Autodesk Fusion 360 part; units mm, degrees
note: some values were not read from the file. Set by a fixed rule: which sketch regions a step uses.
(part 3 of 10)
  spline S13 degree 5 poles (-8.3931, 13.6219) (-8.3929, 13.6198) (-8.3924, 13.6155) (-8.3916, 13.6092) (-8.3906, 13.6008) (-8.3893, 13.5903) (-8.3879, 13.5798) (-8.3866, 13.5693) (-8.3853, 13.5589) (-8.3839, 13.5485) (-8.3826, 13.5382) (-8.3812, 13.5278) (-8.3798, 13.5175) (-8.3784, 13.5072) (-8.377, 13.497) (-8.3755, 13.4867) (-8.3741, 13.4766) (-8.3726, 13.4664) (-8.3712, 13.4563) (-8.3697, 13.4461) (-8.3682, 13.4361) (-8.3667, 13.426) (-8.3652, 13.416) (-8.3637, 13.406) (-8.3621, 13.396) (-8.3606, 13.3861) (-8.359, 13.3762) (-8.3574, 13.3663) (-8.3558, 13.3565) (-8.3542, 13.3467) (-8.3526, 13.3369) (-8.351, 13.3272) (-8.3494, 13.3174) (-8.3477, 13.3078) (-8.3461, 13.2981) (-8.3444, 13.2885) (-8.3427, 13.2789) (-8.341, 13.2693) (-8.3393, 13.2598) (-8.3376, 13.2503) (-8.3359, 13.2408) (-8.3342, 13.2313) (-8.3324, 13.2219) (-8.3307, 13.2125) (-8.3289, 13.2032) (-8.3271, 13.1939) (-8.3254, 13.1846) (-8.3236, 13.1753) (-8.3218, 13.1661) (-8.3199, 13.1569) (-8.3181, 13.1478) (-8.3163, 13.1386) (-8.3145, 13.1296) (-8.3126, 13.1205) (-8.3107, 13.1115) (-8.3089, 13.1025) (-8.307, 13.0935) (-8.3051, 13.0846) (-8.3032, 13.0757) (-8.3013, 13.0668) (-8.2994, 13.058) (-8.2975, 13.0492) (-8.2956, 13.0404) (-8.2936, 13.0317) (-8.2917, 13.023) (-8.2897, 13.0143) (-8.2878, 13.0057) (-8.2858, 12.9971) (-8.2838, 12.9885) (-8.2818, 12.98) (-8.2799, 12.9715) (-8.2779, 12.963) (-8.2759, 12.9546) (-8.2738, 12.9462) (-8.2718, 12.9379) (-8.2698, 12.9295) (-8.2678, 12.9212) (-8.2657, 12.913) (-8.2637, 12.9048) (-8.2616, 12.8966) (-8.2596, 12.8884) (-8.2575, 12.8803) (-8.2554, 12.8722) (-8.2534, 12.8642) (-8.2513, 12.8562) (-8.2492, 12.8482) (-8.2471, 12.8403) (-8.245, 12.8324) (-8.2429, 12.8245) (-8.2408, 12.8167) (-8.2387, 12.8089) (-8.2366, 12.8011) (-8.2345, 12.7934) (-8.2323, 12.7857) (-8.2302, 12.7781) (-8.2281, 12.7705) (-8.2259, 12.7629) (-8.2238, 12.7554) (-8.2216, 12.7479) (-8.2195, 12.7404) (-8.2173, 12.733) (-8.2152, 12.7256) (-8.213, 12.7183) (-8.2109, 12.711) (-8.2087, 12.7037) (-8.2065, 12.6965) (-8.2044, 12.6893) (-8.2022, 12.6821) (-8.2, 12.675) (-8.1978, 12.6679) (-8.1956, 12.6609) (-8.1935, 12.6539) (-8.1913, 12.6469) (-8.1891, 12.64) (-8.1869, 12.6331) (-8.1847, 12.6263) (-8.1825, 12.6195) (-8.1803, 12.6127) (-8.1782, 12.606) (-8.176, 12.5993) (-8.1738, 12.5926) (-8.1716, 12.586) (-8.1694, 12.5795) (-8.1672, 12.5729) (-8.165, 12.5665) (-8.1628, 12.56) (-8.1606, 12.5536) (-8.1584, 12.5473) (-8.1563, 12.5409) (-8.1541, 12.5347) (-8.1519, 12.5284) (-8.1497, 12.5222) (-8.1475, 12.5161) (-8.1453, 12.51) (-8.1432, 12.5039) (-8.141, 12.4979) (-8.1388, 12.4919) (-8.1366, 12.4859) (-8.1345, 12.48) (-8.1323, 12.4742) (-8.1302, 12.4683) (-8.128, 12.4626) (-8.1258, 12.4568) (-8.1237, 12.4512) (-8.1215, 12.4455) (-8.1194, 12.4399) (-8.1173, 12.4344) (-8.1151, 12.4289) (-8.113, 12.4234) (-8.1109, 12.418) (-8.1088, 12.4126) (-8.1067, 12.4073) (-8.1046, 12.402) (-8.1025, 12.3967) (-8.1004, 12.3915) (-8.0983, 12.3864) (-8.0962, 12.3813) (-8.0941, 12.3762) (-8.0921, 12.3712) (-8.09, 12.3662) (-8.088, 12.3613) (-8.0859, 12.3564) (-8.0839, 12.3516) (-8.0819, 12.3468) (-8.0799, 12.3421) (-8.0779, 12.3374) (-8.0759, 12.3327) (-8.0739, 12.3281) (-8.0719, 12.3236) (-8.0699, 12.3191) (-8.068, 12.3146) (-8.066, 12.3102) (-8.0641, 12.3059) (-8.0622, 12.3016) (-8.0603, 12.2973) (-8.0584, 12.2931) (-8.0565, 12.289) (-8.0546, 12.2848) (-8.0527, 12.2808) (-8.0509, 12.2768) (-8.0491, 12.2728) (-8.0472, 12.2689) (-8.0454, 12.265) (-8.0436, 12.2612) (-8.0419, 12.2575) (-8.0401, 12.2538) (-8.0383, 12.2501) (-8.0366, 12.2465) (-8.0349, 12.243) (-8.0332, 12.2395) (-8.0315, 12.236) (-8.0298, 12.2326) (-8.0282, 12.2293) (-8.0265, 12.226) (-8.0249, 12.2228) (-8.0233, 12.2196) (-8.0218, 12.2164) (-8.0202, 12.2134) (-8.0187, 12.2104) (-8.0171, 12.2074) (-8.0156, 12.2045) (-8.0142, 12.2016) (-8.0127, 12.1988) (-8.0113, 12.1961) (-8.0098, 12.1934) (-8.0084, 12.1908) (-8.0071, 12.1882) (-8.0057, 12.1857) (-8.0044, 12.1832) (-8.0031, 12.1808) (-8.0018, 12.1785) (-8.0006, 12.1762) (-7.9994, 12.1739) (-7.9982, 12.1718) (-7.997, 12.1696) (-7.9958, 12.1676) (-7.9947, 12.1656) (-7.9936, 12.1637) (-7.9926, 12.1618) (-7.9915, 12.16) (-7.9905, 12.1582) (-7.9896, 12.1565) (-7.9886, 12.1549) (-7.9877, 12.1533) (-7.9868, 12.1518) (-7.986, 12.1504) (-7.9852, 12.149) (-7.9844, 12.1477) (-7.9836, 12.1464) (-7.9829, 12.1452) (-7.9823, 12.1441) (-7.9816, 12.1431) (-7.981, 12.1421) (-7.9804, 12.1411) (-7.9799, 12.1403) (-7.9794, 12.1395) (-7.979, 12.1388) (-7.9786, 12.1381) (-7.9782, 12.1375) (-7.9779, 12.137) (-7.9776, 12.1365) (-7.9774, 12.1362) (-7.9772, 12.136) (-7.9772, 12.1359) (-7.9771, 12.1359) knots -1 -1 -1 -1 -1 -1 -0.99583333 -0.99166667 -0.9875 -0.98333333 -0.97916667 -0.975 -0.97083333 -0.96666667 -0.9625 -0.95833333 -0.95416667 -0.95 -0.94583333 -0.94166667 -0.9375 -0.93333333 -0.92916667 -0.925 -0.92083333 -0.91666667 -0.9125 -0.90833333 -0.90416667 -0.9 -0.89583333 -0.89166667 -0.8875 -0.88333333 -0.87916667 -0.875 -0.87083333 -0.86666667 -0.8625 -0.85833333 -0.85416667 -0.85 -0.84583333 -0.84166667 -0.8375 -0.83333333 -0.82916667 -0.825 -0.82083333 -0.81666667 -0.8125 -0.80833333 -0.80416667 -0.8 -0.79583333 -0.79166667 -0.7875 -0.78333333 -0.77916667 -0.775 -0.77083333 -0.76666667 -0.7625 -0.75833333 -0.75416667 -0.75 -0.74583333 -0.74166667 -0.7375 -0.73333333 -0.72916667 -0.725 -0.72083333 -0.71666667 -0.7125 -0.70833333 -0.70416667 -0.7 -0.69583333 -0.69166667 -0.6875 -0.68333333 -0.67916667 -0.675 -0.67083333 -0.66666667 -0.6625 -0.65833333 -0.65416667 -0.65 -0.64583333 -0.64166667 -0.6375 -0.63333333 -0.62916667 -0.625 -0.62083333 -0.61666667 -0.6125 -0.60833333 -0.60416667 -0.6 -0.59583333 -0.59166667 -0.5875 -0.58333333 -0.57916667 -0.575 -0.57083333 -0.56666667 -0.5625 -0.55833333 -0.55416667 -0.55 -0.54583333 -0.54166667 -0.5375 -0.53333333 -0.52916667 -0.525 -0.52083333 -0.51666667 -0.5125 -0.50833333 -0.50416667 -0.5 -0.49583333 -0.49166667 -0.4875 -0.48333333 -0.47916667 -0.475 -0.47083333 -0.46666667 -0.4625 -0.45833333 -0.45416667 -0.45 -0.44583333 -0.44166667 -0.4375 -0.43333333 -0.42916667 -0.425 -0.42083333 -0.41666667 -0.4125 -0.40833333 -0.40416667 -0.4 -0.39583333 -0.39166667 -0.3875 -0.38333333 -0.37916667 -0.375 -0.37083333 -0.36666667 -0.3625 -0.35833333 -0.35416667 -0.35 -0.34583333 -0.34166667 -0.3375 -0.33333333 -0.32916667 -0.325 -0.32083333 -0.31666667 -0.3125 -0.30833333 -0.30416667 -0.3 -0.29583333 -0.29166667 -0.2875 -0.28333333 -0.27916667 -0.275 -0.27083333 -0.26666667 -0.2625 -0.25833333 -0.25416667 -0.25 -0.24583333 -0.24166667 -0.2375 -0.23333333 -0.22916667 -0.225 -0.22083333 -0.21666667 -0.2125 -0.20833333 -0.20416667 -0.2 -0.19583333 -0.19166667 -0.1875 -0.18333333 -0.17916667 -0.175 -0.17083333 -0.16666667 -0.1625 -0.15833333 -0.15416667 -0.15 -0.14583333 -0.14166667 -0.1375 -0.13333333 -0.12916667 -0.125 -0.12083333 -0.11666667 -0.1125 -0.10833333 -0.10416667 -0.1 -0.09583333 -0.09166667 -0.0875 -0.08333333 -0.07916667 -0.075 -0.07083333 -0.06666667 -0.0625 -0.05833333 -0.05416667 -0.05 -0.04583333 -0.04166667 -0.0375 -0.03333333 -0.02916667 -0.025 -0.02083333 -0.01666667 -0.0125 -0.00833333 -0.00416667 0 0 0 0 0 0
  line L27 (6.5211, 12.9757) -> (6.1743, 12.2858)
  arc A18 (-13.208, -9.0304) -> (-12.6699, -9.771) centre (0, 0) ccw
  spline S14 degree 5 poles (-9.0768, 11.3369) (-9.0769, 11.3369) (-9.0769, 11.337) (-9.0771, 11.3372) (-9.0773, 11.3375) (-9.0777, 11.3379) (-9.0781, 11.3384) (-9.0785, 11.3389) (-9.079, 11.3395) (-9.0796, 11.3402) (-9.0802, 11.3409) (-9.0808, 11.3417) (-9.0815, 11.3425) (-9.0823, 11.3434) (-9.0831, 11.3443) (-9.084, 11.3453) (-9.0849, 11.3464) (-9.0858, 11.3475) (-9.0868, 11.3486) (-9.0879, 11.3498) (-9.089, 11.3511) (-9.0902, 11.3524) (-9.0914, 11.3537) (-9.0926, 11.3551) (-9.0939, 11.3566) (-9.0953, 11.3581) (-9.0967, 11.3596) (-9.0982, 11.3612) (-9.0997, 11.3628) (-9.1012, 11.3645) (-9.1028, 11.3662) (-9.1045, 11.368) (-9.1062, 11.3698) (-9.1079, 11.3717) (-9.1097, 11.3735) (-9.1115, 11.3755) (-9.1134, 11.3775) (-9.1153, 11.3795) (-9.1173, 11.3815) (-9.1194, 11.3836) (-9.1214, 11.3858) (-9.1235, 11.388) (-9.1257, 11.3902) (-9.1279, 11.3924) (-9.1302, 11.3947) (-9.1325, 11.397) (-9.1348, 11.3994) (-9.1372, 11.4018) (-9.1397, 11.4042) (-9.1422, 11.4067) (-9.1447, 11.4092) (-9.1473, 11.4117) (-9.1499, 11.4143) (-9.1526, 11.4169) (-9.1553, 11.4195) (-9.158, 11.4222) (-9.1608, 11.4249) (-9.1637, 11.4276) (-9.1666, 11.4304) (-9.1695, 11.4332) (-9.1725, 11.436) (-9.1755, 11.4389) (-9.1786, 11.4418) (-9.1817, 11.4447) (-9.1848, 11.4476) (-9.188, 11.4506) (-9.1913, 11.4536) (-9.1946, 11.4566) (-9.1979, 11.4597) (-9.2013, 11.4627) (-9.2047, 11.4658) (-9.2081, 11.469) (-9.2116, 11.4721) (-9.2152, 11.4753) (-9.2188, 11.4785) (-9.2224, 11.4818) (-9.2261, 11.485) (-9.2298, 11.4883) (-9.2335, 11.4916) (-9.2373, 11.495) (-9.2412, 11.4983) (-9.2451, 11.5017) (-9.249, 11.5051) (-9.253, 11.5085) (-9.257, 11.512) (-9.261, 11.5154) (-9.2651, 11.5189) (-9.2692, 11.5224) (-9.2734, 11.526) (-9.2776, 11.5295) (-9.2819, 11.5331) (-9.2862, 11.5367) (-9.2905, 11.5403) (-9.2949, 11.544) (-9.2993, 11.5476) (-9.3038, 11.5513) (-9.3083, 11.555) (-9.3128, 11.5587) (-9.3174, 11.5624) (-9.322, 11.5662) (-9.3267, 11.5699) (-9.3314, 11.5737) (-9.3361, 11.5775) (-9.3409, 11.5813) (-9.3457, 11.5852) (-9.3506, 11.589) (-9.3555, 11.5929) (-9.3605, 11.5968) (-9.3654, 11.6007) (-9.3705, 11.6046) (-9.3755, 11.6085) (-9.3806, 11.6125) (-9.3858, 11.6164) (-9.3909, 11.6204) (-9.3962, 11.6244) (-9.4014, 11.6284) (-9.4067, 11.6324) (-9.412, 11.6365) (-9.4174, 11.6405) (-9.4228, 11.6446) (-9.4283, 11.6486) (-9.4338, 11.6527) (-9.4393, 11.6568) (-9.4449, 11.6609) (-9.4505, 11.6651) (-9.4561, 11.6692) (-9.4618, 11.6733) (-9.4675, 11.6775) (-9.4733, 11.6817) (-9.4791, 11.6859) (-9.4849, 11.6901) (-9.4908, 11.6943) (-9.4967, 11.6985) (-9.5026, 11.7027) (-9.5086, 11.707) (-9.5146, 11.7112) (-9.5207, 11.7155) (-9.5268, 11.7197) (-9.5329, 11.724) (-9.5391, 11.7283) (-9.5453, 11.7326) (-9.5516, 11.7369) (-9.5578, 11.7412) (-9.5642, 11.7455) (-9.5705, 11.7499) (-9.5769, 11.7542) (-9.5833, 11.7586) (-9.5898, 11.7629) (-9.5963, 11.7673) (-9.6028, 11.7717) (-9.6094, 11.776) (-9.616, 11.7804) (-9.6227, 11.7848) (-9.6294, 11.7892) (-9.6361, 11.7936) (-9.6428, 11.798) (-9.6496, 11.8025) (-9.6565, 11.8069) (-9.6633, 11.8113) (-9.6702, 11.8158) (-9.6772, 11.8202) (-9.6841, 11.8247) (-9.6912, 11.8291) (-9.6982, 11.8336) (-9.7053, 11.8381) (-9.7124, 11.8425) (-9.7195, 11.847) (-9.7267, 11.8515) (-9.7339, 11.856) (-9.7412, 11.8605) (-9.7485, 11.865) (-9.7558, 11.8695) (-9.7632, 11.874) (-9.7706, 11.8785) (-9.778, 11.883) (-9.7855, 11.8875) (-9.793, 11.8921) (-9.8005, 11.8966) (-9.8081, 11.9011) (-9.8157, 11.9056) (-9.8233, 11.9102) (-9.831, 11.9147) (-9.8387, 11.9193) (-9.8464, 11.9238) (-9.8542, 11.9283) (-9.862, 11.9329) (-9.8699, 11.9374) (-9.8777, 11.942) (-9.8857, 11.9465) (-9.8936, 11.9511) (-9.9016, 11.9557) (-9.9096, 11.9602) (-9.9176, 11.9648) (-9.9257, 11.9693) (-9.9338, 11.9739) (-9.942, 11.9785) (-9.9502, 11.983) (-9.9584, 11.9876) (-9.9666, 11.9921) (-9.9749, 11.9967) (-9.9832, 12.0013) (-9.9916, 12.0058) (-9.9999, 12.0104) (-10.0084, 12.015) (-10.0168, 12.0195) (-10.0253, 12.0241) (-10.0338, 12.0287) (-10.0423, 12.0332) (-10.0509, 12.0378) (-10.0595, 12.0423) (-10.0682, 12.0469) (-10.0768, 12.0515) (-10.0855, 12.056) (-10.0943, 12.0606) (-10.1031, 12.0651) (-10.1119, 12.0697) (-10.1207, 12.0743) (-10.1296, 12.0788) (-10.1385, 12.0834) (-10.1474, 12.0879) (-10.1564, 12.0924) (-10.1654, 12.097) (-10.1744, 12.1015) (-10.1834, 12.1061) (-10.1925, 12.1106) (-10.2017, 12.1151) (-10.2108, 12.1197) (-10.22, 12.1242) (-10.2292, 12.1287) (-10.2385, 12.1332) (-10.2478, 12.1378) (-10.2571, 12.1423) (-10.2664, 12.1468) (-10.2758, 12.1513) (-10.2852, 12.1558) (-10.2946, 12.1603) (-10.3041, 12.1648) (-10.3136, 12.1693) (-10.3231, 12.1738) (-10.3327, 12.1783) (-10.3423, 12.1828) (-10.35, 12.1863) (-10.3558, 12.189) (-10.3596, 12.1908) (-10.3616, 12.1917) knots 0 0 0 0 0 0 0.00416667 0.00833333 0.0125 0.01666667 0.02083333 0.025 0.02916667 0.03333333 0.0375 0.04166667 0.04583333 0.05 0.05416667 0.05833333 0.0625 0.06666667 0.07083333 0.075 0.07916667 0.08333333 0.0875 0.09166667 0.09583333 0.1 0.10416667 0.10833333 0.1125 0.11666667 0.12083333 0.125 0.12916667 0.13333333 0.1375 0.14166667 0.14583333 0.15 0.15416667 0.15833333 0.1625 0.16666667 0.17083333 0.175 0.17916667 0.18333333 0.1875 0.19166667 0.19583333 0.2 0.20416667 0.20833333 0.2125 0.21666667 0.22083333 0.225 0.22916667 0.23333333 0.2375 0.24166667 0.24583333 0.25 0.25416667 0.25833333 0.2625 0.26666667 0.27083333 0.275 0.27916667 0.28333333 0.2875 0.29166667 0.29583333 0.3 0.30416667 0.30833333 0.3125 0.31666667 0.32083333 0.325 0.32916667 0.33333333 0.3375 0.34166667 0.34583333 0.35 0.35416667 0.35833333 0.3625 0.36666667 0.37083333 0.375 0.37916667 0.38333333 0.3875 0.39166667 0.39583333 0.4 0.40416667 0.40833333 0.4125 0.41666667 0.42083333 0.425 0.42916667 0.43333333 0.4375 0.44166667 0.44583333 0.45 0.45416667 0.45833333 0.4625 0.46666667 0.47083333 0.475 0.47916667 0.48333333 0.4875 0.49166667 0.49583333 0.5 0.50416667 0.50833333 0.5125 0.51666667 0.52083333 0.525 0.52916667 0.53333333 0.5375 0.54166667 0.54583333 0.55 0.55416667 0.55833333 0.5625 0.56666667 0.57083333 0.575 0.57916667 0.58333333 0.5875 0.59166667 0.59583333 0.6 0.60416667 0.60833333 0.6125 0.61666667 0.62083333 0.625 0.62916667 0.63333333 0.6375 0.64166667 0.64583333 0.65 0.65416667 0.65833333 0.6625 0.66666667 0.67083333 0.675 0.67916667 0.68333333 0.6875 0.69166667 0.69583333 0.7 0.70416667 0.70833333 0.7125 0.71666667 0.72083333 0.725 0.72916667 0.73333333 0.7375 0.74166667 0.74583333 0.75 0.75416667 0.75833333 0.7625 0.76666667 0.77083333 0.775 0.77916667 0.78333333 0.7875 0.79166667 0.79583333 0.8 0.80416667 0.80833333 0.8125 0.81666667 0.82083333 0.825 0.82916667 0.83333333 0.8375 0.84166667 0.84583333 0.85 0.85416667 0.85833333 0.8625 0.86666667 0.87083333 0.875 0.87916667 0.88333333 0.8875 0.89166667 0.89583333 0.9 0.90416667 0.90833333 0.9125 0.91666667 0.92083333 0.925 0.92916667 0.93333333 0.9375 0.94166667 0.94583333 0.95 0.95416667 0.95833333 0.9625 0.96666667 0.97083333 0.975 0.97916667 0.98333333 0.9875 0.99166667 0.99583333 1 1 1 1 1 1
  spline S15 degree 5 poles (-13.208, 9.0304) (-13.2069, 9.0286) (-13.2047, 9.0249) (-13.2015, 9.0195) (-13.1971, 9.0122) (-13.1916, 9.0031) (-13.1862, 8.9941) (-13.1807, 8.9851) (-13.1752, 8.9761) (-13.1698, 8.9671) (-13.1643, 8.9582) (-13.1589, 8.9493) (-13.1534, 8.9405) (-13.1479, 8.9317) (-13.1425, 8.9229) (-13.137, 8.9141) (-13.1315, 8.9054) (-13.1261, 8.8967) (-13.1206, 8.888) (-13.1151, 8.8794) (-13.1097, 8.8708) (-13.1042, 8.8622) (-13.0988, 8.8537) (-13.0933, 8.8452) (-13.0878, 8.8367) (-13.0824, 8.8283) (-13.0769, 8.8199) (-13.0715, 8.8115) (-13.066, 8.8032) (-13.0606, 8.7948) (-13.0551, 8.7866) (-13.0497, 8.7783) (-13.0442, 8.7701) (-13.0388, 8.7619) (-13.0333, 8.7538) (-13.0279, 8.7456) (-13.0224, 8.7376) (-13.017, 8.7295) (-13.0116, 8.7215) (-13.0062, 8.7135) (-13.0007, 8.7055) (-12.9953, 8.6976) (-12.9899, 8.6897) (-12.9845, 8.6819) (-12.9791, 8.6741) (-12.9736, 8.6663) (-12.9682, 8.6585) (-12.9628, 8.6508) (-12.9574, 8.6431) (-12.9521, 8.6354) (-12.9467, 8.6278) (-12.9413, 8.6202) (-12.9359, 8.6126) (-12.9305, 8.6051) (-12.9252, 8.5976) (-12.9198, 8.5902) (-12.9144, 8.5827) (-12.9091, 8.5754) (-12.9037, 8.568) (-12.8984, 8.5607) (-12.893, 8.5534) (-12.8877, 8.5461) (-12.8824, 8.5389) (-12.8771, 8.5317) (-12.8718, 8.5246) (-12.8664, 8.5174) (-12.8611, 8.5103) (-12.8558, 8.5033) (-12.8506, 8.4963) (-12.8453, 8.4893) (-12.84, 8.4823) (-12.8347, 8.4754) (-12.8295, 8.4685) (-12.8242, 8.4617) (-12.819, 8.4549) (-12.8138, 8.4481) (-12.8085, 8.4413) (-12.8033, 8.4346) (-12.7981, 8.4279) (-12.7929, 8.4213) (-12.7877, 8.4147) (-12.7825, 8.4081) (-12.7773, 8.4016) (-12.7722, 8.3951) (-12.767, 8.3886) (-12.7619, 8.3822) (-12.7567, 8.3758) (-12.7516, 8.3694) (-12.7465, 8.3631) (-12.7414, 8.3568) (-12.7363, 8.3505) (-12.7312, 8.3443) (-12.7261, 8.3381) (-12.721, 8.332) (-12.716, 8.3259) (-12.7109, 8.3198) (-12.7059, 8.3137) (-12.7009, 8.3077) (-12.6959, 8.3017) (-12.6909, 8.2958) (-12.6859, 8.2899) (-12.6809, 8.284) (-12.676, 8.2782) (-12.671, 8.2724) (-12.6661, 8.2666) (-12.6612, 8.2609) (-12.6562, 8.2552) (-12.6513, 8.2496) (-12.6465, 8.2439) (-12.6416, 8.2384) (-12.6367, 8.2328) (-12.6319, 8.2273) (-12.6271, 8.2218) (-12.6223, 8.2164) (-12.6175, 8.211) (-12.6127, 8.2056) (-12.6079, 8.2003) (-12.6032, 8.195) (-12.5984, 8.1898) (-12.5937, 8.1846) (-12.589, 8.1794) (-12.5843, 8.1742) (-12.5796, 8.1691) (-12.575, 8.1641) (-12.5703, 8.159) (-12.5657, 8.154) (-12.5611, 8.1491) (-12.5565, 8.1441) (-12.552, 8.1393) (-12.5474, 8.1344) (-12.5429, 8.1296) (-12.5384, 8.1248) (-12.5339, 8.1201) (-12.5294, 8.1154) (-12.5249, 8.1107) (-12.5205, 8.1061) (-12.5161, 8.1015) (-12.5117, 8.097) (-12.5073, 8.0925) (-12.5029, 8.088) (-12.4986, 8.0836) (-12.4943, 8.0792) (-12.49, 8.0748) (-12.4857, 8.0705) (-12.4815, 8.0662) (-12.4772, 8.062) (-12.473, 8.0578) (-12.4688, 8.0536) (-12.4647, 8.0495) (-12.4605, 8.0454) (-12.4564, 8.0413) (-12.4523, 8.0373) (-12.4482, 8.0333) (-12.4442, 8.0294) (-12.4401, 8.0255) (-12.4361, 8.0216) (-12.4322, 8.0178) (-12.4282, 8.014) (-12.4243, 8.0103) (-12.4204, 8.0066) (-12.4165, 8.0029) (-12.4127, 7.9993) (-12.4089, 7.9957) (-12.4051, 7.9922) (-12.4013, 7.9887) (-12.3976, 7.9852) (-12.3938, 7.9818) (-12.3902, 7.9784) (-12.3865, 7.975) (-12.3829, 7.9717) (-12.3793, 7.9684) (-12.3757, 7.9652) (-12.3722, 7.962) (-12.3687, 7.9589) (-12.3652, 7.9558) (-12.3617, 7.9527) (-12.3583, 7.9496) (-12.3549, 7.9467) (-12.3516, 7.9437) (-12.3483, 7.9408) (-12.345, 7.9379) (-12.3417, 7.9351) (-12.3385, 7.9323) (-12.3353, 7.9296) (-12.3322, 7.9268) (-12.329, 7.9242) (-12.326, 7.9216) (-12.3229, 7.919) (-12.3199, 7.9164) (-12.3169, 7.9139) (-12.314, 7.9115) (-12.3111, 7.909) (-12.3082, 7.9066) (-12.3054, 7.9043) (-12.3026, 7.902) (-12.2998, 7.8998) (-12.2971, 7.8975) (-12.2944, 7.8954) (-12.2918, 7.8932) (-12.2892, 7.8911) (-12.2867, 7.8891) (-12.2841, 7.8871) (-12.2817, 7.8851) (-12.2792, 7.8832) (-12.2769, 7.8813) (-12.2745, 7.8795) (-12.2722, 7.8777) (-12.27, 7.8759) (-12.2677, 7.8742) (-12.2656, 7.8726) (-12.2635, 7.8709) (-12.2614, 7.8693) (-12.2594, 7.8678) (-12.2574, 7.8663) (-12.2555, 7.8649) (-12.2536, 7.8634) (-12.2517, 7.8621) (-12.25, 7.8608) (-12.2482, 7.8595) (-12.2465, 7.8582) (-12.2449, 7.857) (-12.2433, 7.8559) (-12.2418, 7.8548) (-12.2403, 7.8537) (-12.2389, 7.8527) (-12.2376, 7.8517) (-12.2363, 7.8508) (-12.235, 7.8499) (-12.2338, 7.8491) (-12.2327, 7.8483) (-12.2316, 7.8475) (-12.2306, 7.8468) (-12.2296, 7.8462) (-12.2287, 7.8455) (-12.2279, 7.845) (-12.2271, 7.8445) (-12.2264, 7.844) (-12.2258, 7.8435) (-12.2252, 7.8431) (-12.2247, 7.8428) (-12.2242, 7.8425) (-12.2239, 7.8423) (-12.2237, 7.8422) (-12.2236, 7.8421) (-12.2236, 7.8421) knots -1 -1 -1 -1 -1 -1 -0.99583333 -0.99166667 -0.9875 -0.98333333 -0.97916667 -0.975 -0.97083333 -0.96666667 -0.9625 -0.95833333 -0.95416667 -0.95 -0.94583333 -0.94166667 -0.9375 -0.93333333 -0.92916667 -0.925 -0.92083333 -0.91666667 -0.9125 -0.90833333 -0.90416667 -0.9 -0.89583333 -0.89166667 -0.8875 -0.88333333 -0.87916667 -0.875 -0.87083333 -0.86666667 -0.8625 -0.85833333 -0.85416667 -0.85 -0.84583333 -0.84166667 -0.8375 -0.83333333 -0.82916667 -0.825 -0.82083333 -0.81666667 -0.8125 -0.80833333 -0.80416667 -0.8 -0.79583333 -0.79166667 -0.7875 -0.78333333 -0.77916667 -0.775 -0.77083333 -0.76666667 -0.7625 -0.75833333 -0.75416667 -0.75 -0.74583333 -0.74166667 -0.7375 -0.73333333 -0.72916667 -0.725 -0.72083333 -0.71666667 -0.7125 -0.70833333 -0.70416667 -0.7 -0.69583333 -0.69166667 -0.6875 -0.68333333 -0.67916667 -0.675 -0.67083333 -0.66666667 -0.6625 -0.65833333 -0.65416667 -0.65 -0.64583333 -0.64166667 -0.6375 -0.63333333 -0.62916667 -0.625 -0.62083333 -0.61666667 -0.6125 -0.60833333 -0.60416667 -0.6 -0.59583333 -0.59166667 -0.5875 -0.58333333 -0.57916667 -0.575 -0.57083333 -0.56666667 -0.5625 -0.55833333 -0.55416667 -0.55 -0.54583333 -0.54166667 -0.5375 -0.53333333 -0.52916667 -0.525 -0.52083333 -0.51666667 -0.5125 -0.50833333 -0.50416667 -0.5 -0.49583333 -0.49166667 -0.4875 -0.48333333 -0.47916667 -0.475 -0.47083333 -0.46666667 -0.4625 -0.45833333 -0.45416667 -0.45 -0.44583333 -0.44166667 -0.4375 -0.43333333 -0.42916667 -0.425 -0.42083333 -0.41666667 -0.4125 -0.40833333 -0.40416667 -0.4 -0.39583333 -0.39166667 -0.3875 -0.38333333 -0.37916667 -0.375 -0.37083333 -0.36666667 -0.3625 -0.35833333 -0.35416667 -0.35 -0.34583333 -0.34166667 -0.3375 -0.33333333 -0.32916667 -0.325 -0.32083333 -0.31666667 -0.3125 -0.30833333 -0.30416667 -0.3 -0.29583333 -0.29166667 -0.2875 -0.28333333 -0.27916667 -0.275 -0.27083333 -0.26666667 -0.2625 -0.25833333 -0.25416667 -0.25 -0.24583333 -0.24166667 -0.2375 -0.23333333 -0.22916667 -0.225 -0.22083333 -0.21666667 -0.2125 -0.20833333 -0.20416667 -0.2 -0.19583333 -0.19166667 -0.1875 -0.18333333 -0.17916667 -0.175 -0.17083333 -0.16666667 -0.1625 -0.15833333 -0.15416667 -0.15 -0.14583333 -0.14166667 -0.1375 -0.13333333 -0.12916667 -0.125 -0.12083333 -0.11666667 -0.1125 -0.10833333 -0.10416667 -0.1 -0.09583333 -0.09166667 -0.0875 -0.08333333 -0.07916667 -0.075 -0.07083333 -0.06666667 -0.0625 -0.05833333 -0.05416667 -0.05 -0.04583333 -0.04166667 -0.0375 -0.03333333 -0.02916667 -0.025 -0.02083333 -0.01666667 -0.0125 -0.00833333 -0.00416667 0 0 0 0 0 0
  line L28 (-10.3255, -10.2117) -> (-10.326, -10.2121)
  line L29 (-8.5938, 10.7336) -> (-9.0764, 11.3364)
  arc A19 (-9.7765, 9.6687) -> (-10.6376, 8.7123) centre (0, 0) ccw
  line L30 (-9.0768, -11.3369) -> (-9.0764, -11.3364)
  arc A20 (-10.3616, 12.1917) -> (-11.0419, 11.5792) centre (0, 0) ccw
  line L31 (-10.6376, 8.7123) -> (-11.235, 9.2016)
  arc A21 (-12.6699, 9.771) -> (-13.208, 9.0304) centre (0, 0) ccw
  line L32 (-7.5526, -11.49) -> (-7.9768, -12.1353)
  line L33 (-9.0764, -11.3364) -> (-8.5938, -10.7336)
  line L34 (-5.2796, 13.5292) -> (-5.2794, 13.5286)
  line L35 (-10.3255, 10.2117) -> (-9.7765, 9.6687)
  line L36 (3.6808, 14.048) -> (3.4851, 13.301)
  line L37 (-0.6435, 13.7349) -> (-0.6796, 14.5063)
  line L38 (-6.1743, 12.2858) -> (-6.5211, 12.9757)
  line L39 (-2.3514, 14.3312) -> (-2.3513, 14.3306)
  line L40 (2.2262, 13.5686) -> (2.3513, 14.3306)
  line L41 (-3.4851, 13.301) -> (-3.6808, 14.048)
  line L42 (-3.6808, 14.048) -> (-3.681, 14.0486)
  line L43 (-2.3513, 14.3306) -> (-2.2262, 13.5686)
  line L44 (-0.6796, 14.5063) -> (-0.6796, 14.5069)
  line L45 (-7.9771, 12.1359) -> (-7.9768, 12.1353)
  line L46 (-6.5211, 12.9757) -> (-6.5214, 12.9763)
  arc A22 (-8.3931, -13.6219) -> (-7.6003, -14.0796) centre (0, 0) ccw
  line L47 (-7.9768, 12.1353) -> (-7.5526, 11.49)
  line L48 (5.2794, 13.5286) -> (5.2796, 13.5292)
  arc A23 (-8.5938, -10.7336) -> (-7.5526, -11.49) centre (0, 0) ccw
  line L49 (-10.326, 10.2121) -> (-10.3255, 10.2117)
  line L50 (3.681, 14.0486) -> (3.6808, 14.048)
  spline S16 degree 5 poles (-12.2236, -7.8421) (-12.2236, -7.8421) (-12.2237, -7.8422) (-12.2239, -7.8423) (-12.2242, -7.8425) (-12.2247, -7.8428) (-12.2252, -7.8431) (-12.2258, -7.8435) (-12.2264, -7.844) (-12.2271, -7.8445) (-12.2279, -7.845) (-12.2287, -7.8455) (-12.2296, -7.8462) (-12.2306, -7.8468) (-12.2316, -7.8475) (-12.2327, -7.8483) (-12.2338, -7.8491) (-12.235, -7.8499) (-12.2363, -7.8508) (-12.2376, -7.8517) (-12.2389, -7.8527) (-12.2403, -7.8537) (-12.2418, -7.8548) (-12.2433, -7.8559) (-12.2449, -7.857) (-12.2465, -7.8582) (-12.2482, -7.8595) (-12.25, -7.8608) (-12.2517, -7.8621) (-12.2536, -7.8634) (-12.2555, -7.8649) (-12.2574, -7.8663) (-12.2594, -7.8678) (-12.2614, -7.8693) (-12.2635, -7.8709) (-12.2656, -7.8726) (-12.2677, -7.8742) (-12.27, -7.8759) (-12.2722, -7.8777) (-12.2745, -7.8795) (-12.2769, -7.8813) (-12.2792, -7.8832) (-12.2817, -7.8851) (-12.2841, -7.8871) (-12.2867, -7.8891) (-12.2892, -7.8911) (-12.2918, -7.8932) (-12.2944, -7.8954) (-12.2971, -7.8975) (-12.2998, -7.8998) (-12.3026, -7.902) (-12.3054, -7.9043) (-12.3082, -7.9066) (-12.3111, -7.909) (-12.314, -7.9115) (-12.3169, -7.9139) (-12.3199, -7.9164) (-12.3229, -7.919) (-12.326, -7.9216) (-12.329, -7.9242) (-12.3322, -7.9268) (-12.3353, -7.9296) (-12.3385, -7.9323) (-12.3417, -7.9351) (-12.345, -7.9379) (-12.3483, -7.9408) (-12.3516, -7.9437) (-12.3549, -7.9467) (-12.3583, -7.9496) (-12.3617, -7.9527) (-12.3652, -7.9558) (-12.3687, -7.9589) (-12.3722, -7.962) (-12.3757, -7.9652) (-12.3793, -7.9684) (-12.3829, -7.9717) (-12.3865, -7.975) (-12.3902, -7.9784) (-12.3938, -7.9818) (-12.3976, -7.9852) (-12.4013, -7.9887) (-12.4051, -7.9922) (-12.4089, -7.9957) (-12.4127, -7.9993) (-12.4165, -8.0029) (-12.4204, -8.0066) (-12.4243, -8.0103) (-12.4282, -8.014) (-12.4322, -8.0178) (-12.4361, -8.0216) (-12.4401, -8.0255) (-12.4442, -8.0294) (-12.4482, -8.0333) (-12.4523, -8.0373) (-12.4564, -8.0413) (-12.4605, -8.0454) (-12.4647, -8.0495) (-12.4688, -8.0536) (-12.473, -8.0578) (-12.4772, -8.062) (-12.4815, -8.0662) (-12.4857, -8.0705) (-12.49, -8.0748) (-12.4943, -8.0792) (-12.4986, -8.0836) (-12.5029, -8.088) (-12.5073, -8.0925) (-12.5117, -8.097) (-12.5161, -8.1015) (-12.5205, -8.1061) (-12.5249, -8.1107) (-12.5294, -8.1154) (-12.5339, -8.1201) (-12.5384, -8.1248) (-12.5429, -8.1296) (-12.5474, -8.1344) (-12.552, -8.1393) (-12.5565, -8.1441) (-12.5611, -8.1491) (-12.5657, -8.154) (-12.5703, -8.159) (-12.575, -8.1641) (-12.5796, -8.1691) (-12.5843, -8.1742) (-12.589, -8.1794) (-12.5937, -8.1846) (-12.5984, -8.1898) (-12.6032, -8.195) (-12.6079, -8.2003) (-12.6127, -8.2056) (-12.6175, -8.211) (-12.6223, -8.2164) (-12.6271, -8.2218) (-12.6319, -8.2273) (-12.6367, -8.2328) (-12.6416, -8.2384) (-12.6465, -8.2439) (-12.6513, -8.2496) (-12.6562, -8.2552) (-12.6612, -8.2609) (-12.6661, -8.2666) (-12.671, -8.2724) (-12.676, -8.2782) (-12.6809, -8.284) (-12.6859, -8.2899) (-12.6909, -8.2958) (-12.6959, -8.3017) (-12.7009, -8.3077) (-12.7059, -8.3137) (-12.7109, -8.3198) (-12.716, -8.3259) (-12.721, -8.332) (-12.7261, -8.3381) (-12.7312, -8.3443) (-12.7363, -8.3505) (-12.7414, -8.3568) (-12.7465, -8.3631) (-12.7516, -8.3694) (-12.7567, -8.3758) (-12.7619, -8.3822) (-12.767, -8.3886) (-12.7722, -8.3951) (-12.7773, -8.4016) (-12.7825, -8.4081) (-12.7877, -8.4147) (-12.7929, -8.4213) (-12.7981, -8.4279) (-12.8033, -8.4346) (-12.8085, -8.4413) (-12.8138, -8.4481) (-12.819, -8.4549) (-12.8242, -8.4617) (-12.8295, -8.4685) (-12.8347, -8.4754) (-12.84, -8.4823) (-12.8453, -8.4893) (-12.8506, -8.4963) (-12.8558, -8.5033) (-12.8611, -8.5103) (-12.8664, -8.5174) (-12.8718, -8.5246) (-12.8771, -8.5317) (-12.8824, -8.5389) (-12.8877, -8.5461) (-12.893, -8.5534) (-12.8984, -8.5607) (-12.9037, -8.568) (-12.9091, -8.5754) (-12.9144, -8.5827) (-12.9198, -8.5902) (-12.9252, -8.5976) (-12.9305, -8.6051) (-12.9359, -8.6126) (-12.9413, -8.6202) (-12.9467, -8.6278) (-12.9521, -8.6354) (-12.9574, -8.6431) (-12.9628, -8.6508) (-12.9682, -8.6585) (-12.9736, -8.6663) (-12.9791, -8.6741) (-12.9845, -8.6819) (-12.9899, -8.6897) (-12.9953, -8.6976) (-13.0007, -8.7055) (-13.0062, -8.7135) (-13.0116, -8.7215) (-13.017, -8.7295) (-13.0224, -8.7376) (-13.0279, -8.7456) (-13.0333, -8.7538) (-13.0388, -8.7619) (-13.0442, -8.7701) (-13.0497, -8.7783) (-13.0551, -8.7866) (-13.0606, -8.7948) (-13.066, -8.8032) (-13.0715, -8.8115) (-13.0769, -8.8199) (-13.0824, -8.8283) (-13.0878, -8.8367) (-13.0933, -8.8452) (-13.0988, -8.8537) (-13.1042, -8.8622) (-13.1097, -8.8708) (-13.1151, -8.8794) (-13.1206, -8.888) (-13.1261, -8.8967) (-13.1315, -8.9054) (-13.137, -8.9141) (-13.1425, -8.9229) (-13.1479, -8.9317) (-13.1534, -8.9405) (-13.1589, -8.9493) (-13.1643, -8.9582) (-13.1698, -8.9671) (-13.1752, -8.9761) (-13.1807, -8.9851) (-13.1862, -8.9941) (-13.1916, -9.0031) (-13.1971, -9.0122) (-13.2015, -9.0195) (-13.2047, -9.0249) (-13.2069, -9.0286) (-13.208, -9.0304) knots 0 0 0 0 0 0 0.00416667 0.00833333 0.0125 0.01666667 0.02083333 0.025 0.02916667 0.03333333 0.0375 0.04166667 0.04583333 0.05 0.05416667 0.05833333 0.0625 0.06666667 0.07083333 0.075 0.07916667 0.08333333 0.0875 0.09166667 0.09583333 0.1 0.10416667 0.10833333 0.1125 0.11666667 0.12083333 0.125 0.12916667 0.13333333 0.1375 0.14166667 0.14583333 0.15 0.15416667 0.15833333 0.1625 0.16666667 0.17083333 0.175 0.17916667 0.18333333 0.1875 0.19166667 0.19583333 0.2 0.20416667 0.20833333 0.2125 0.21666667 0.22083333 0.225 0.22916667 0.23333333 0.2375 0.24166667 0.24583333 0.25 0.25416667 0.25833333 0.2625 0.26666667 0.27083333 0.275 0.27916667 0.28333333 0.2875 0.29166667 0.29583333 0.3 0.30416667 0.30833333 0.3125 0.31666667 0.32083333 0.325 0.32916667 0.33333333 0.3375 0.34166667 0.34583333 0.35 0.35416667 0.35833333 0.3625 0.36666667 0.37083333 0.375 0.37916667 0.38333333 0.3875 0.39166667 0.39583333 0.4 0.40416667 0.40833333 0.4125 0.41666667 0.42083333 0.425 0.42916667 0.43333333 0.4375 0.44166667 0.44583333 0.45 0.45416667 0.45833333 0.4625 0.46666667 0.47083333 0.475 0.47916667 0.48333333 0.4875 0.49166667 0.49583333 0.5 0.50416667 0.50833333 0.5125 0.51666667 0.52083333 0.525 0.52916667 0.53333333 0.5375 0.54166667 0.54583333 0.55 0.55416667 0.55833333 0.5625 0.56666667 0.57083333 0.575 0.57916667 0.58333333 0.5875 0.59166667 0.59583333 0.6 0.60416667 0.60833333 0.6125 0.61666667 0.62083333 0.625 0.62916667 0.63333333 0.6375 0.64166667 0.64583333 0.65 0.65416667 0.65833333 0.6625 0.66666667 0.67083333 0.675 0.67916667 0.68333333 0.6875 0.69166667 0.69583333 0.7 0.70416667 0.70833333 0.7125 0.71666667 0.72083333 0.725 0.72916667 0.73333333 0.7375 0.74166667 0.74583333 0.75 0.75416667 0.75833333 0.7625 0.76666667 0.77083333 0.775 0.77916667 0.78333333 0.7875 0.79166667 0.79583333 0.8 0.80416667 0.80833333 0.8125 0.81666667 0.82083333 0.825 0.82916667 0.83333333 0.8375 0.84166667 0.84583333 0.85 0.85416667 0.85833333 0.8625 0.86666667 0.87083333 0.875 0.87916667 0.88333333 0.8875 0.89166667 0.89583333 0.9 0.90416667 0.90833333 0.9125 0.91666667 0.92083333 0.925 0.92916667 0.93333333 0.9375 0.94166667 0.94583333 0.95 0.95416667 0.95833333 0.9625 0.96666667 0.97083333 0.975 0.97916667 0.98333333 0.9875 0.99166667 0.99583333 1 1 1 1 1 1
  line L51 (3.4851, -13.301) -> (3.6808, -14.048)
  line L52 (9.0764, 11.3364) -> (8.5938, 10.7336)
  line L53 (2.3514, -14.3312) -> (2.3513, -14.3306)
  spline S17 degree 5 poles (-1.2166, -15.9537) (-1.2155, -15.9518) (-1.2135, -15.9481) (-1.2104, -15.9425) (-1.2062, -15.9351) (-1.2011, -15.9258) (-1.196, -15.9166) (-1.1909, -15.9074) (-1.1859, -15.8981) (-1.1809, -15.8889) (-1.1759, -15.8797) (-1.1709, -15.8706) (-1.166, -15.8614) (-1.1611, -15.8523) (-1.1562, -15.8431) (-1.1514, -15.834) (-1.1465, -15.8249) (-1.1417, -15.8159) (-1.137, -15.8068) (-1.1322, -15.7977) (-1.1275, -15.7887) (-1.1228, -15.7797) (-1.1182, -15.7707) (-1.1135, -15.7617) (-1.1089, -15.7528) (-1.1043, -15.7438) (-1.0998, -15.7349) (-1.0952, -15.726) (-1.0907, -15.7171) (-1.0863, -15.7082) (-1.0818, -15.6993) (-1.0774, -15.6905) (-1.073, -15.6817) (-1.0687, -15.6729) (-1.0643, -15.6641) (-1.06, -15.6553) (-1.0557, -15.6466) (-1.0515, -15.6378) (-1.0472, -15.6291) (-1.043, -15.6204) (-1.0389, -15.6117) (-1.0347, -15.6031) (-1.0306, -15.5944) (-1.0265, -15.5858) (-1.0224, -15.5772) (-1.0184, -15.5686) (-1.0144, -15.5601) (-1.0104, -15.5515) (-1.0064, -15.543) (-1.0025, -15.5345) (-0.9986, -15.526) (-0.9947, -15.5176) (-0.9908, -15.5091) (-0.987, -15.5007) (-0.9832, -15.4923) (-0.9794, -15.484) (-0.9757, -15.4756) (-0.9719, -15.4673) (-0.9682, -15.459) (-0.9646, -15.4507) (-0.9609, -15.4424) (-0.9573, -15.4341) (-0.9537, -15.4259) (-0.9501, -15.4177) (-0.9466, -15.4095) (-0.9431, -15.4014) (-0.9396, -15.3932) (-0.9361, -15.3851) (-0.9327, -15.377) (-0.9293, -15.369) (-0.9259, -15.3609) (-0.9225, -15.3529) (-0.9192, -15.3449) (-0.9159, -15.3369) (-0.9126, -15.329) (-0.9094, -15.3211) (-0.9061, -15.3132) (-0.9029, -15.3053) (-0.8998, -15.2974) (-0.8966, -15.2896) (-0.8935, -15.2818) (-0.8904, -15.274) (-0.8873, -15.2663) (-0.8843, -15.2586) (-0.8812, -15.2509) (-0.8782, -15.2432) (-0.8753, -15.2355) (-0.8723, -15.2279) (-0.8694, -15.2203) (-0.8665, -15.2127) (-0.8636, -15.2052) (-0.8608, -15.1977) (-0.858, -15.1902) (-0.8552, -15.1827) (-0.8524, -15.1753) (-0.8497, -15.1679) (-0.8469, -15.1605) (-0.8442, -15.1531) (-0.8416, -15.1458) (-0.8389, -15.1385) (-0.8363, -15.1313) (-0.8337, -15.124) (-0.8311, -15.1168) (-0.8286, -15.1096) (-0.8261, -15.1025) (-0.8236, -15.0953) (-0.8211, -15.0882) (-0.8187, -15.0812) (-0.8162, -15.0741) (-0.8138, -15.0671) (-0.8115, -15.0601) (-0.8091, -15.0532) (-0.8068, -15.0463) (-0.8045, -15.0394) (-0.8022, -15.0325) (-0.8, -15.0257) (-0.7977, -15.0189) (-0.7955, -15.0122) (-0.7933, -15.0054) (-0.7912, -14.9987) (-0.789, -14.9921) (-0.7869, -14.9855) (-0.7848, -14.9789) (-0.7828, -14.9723) (-0.7807, -14.9658) (-0.7787, -14.9593) (-0.7767, -14.9528) (-0.7748, -14.9464) (-0.7728, -14.94) (-0.7709, -14.9336) (-0.769, -14.9273) (-0.7671, -14.921) (-0.7653, -14.9147) (-0.7634, -14.9085) (-0.7616, -14.9023) (-0.7599, -14.8961) (-0.7581, -14.89) (-0.7564, -14.8839) (-0.7546, -14.8779) (-0.7529, -14.8719) (-0.7513, -14.8659) (-0.7496, -14.86) (-0.748, -14.854) (-0.7464, -14.8482) (-0.7448, -14.8424) (-0.7433, -14.8366) (-0.7417, -14.8308) (-0.7402, -14.8251) (-0.7387, -14.8194) (-0.7372, -14.8138) (-0.7358, -14.8082) (-0.7344, -14.8027) (-0.733, -14.7971) (-0.7316, -14.7917) (-0.7302, -14.7862) (-0.7289, -14.7808) (-0.7276, -14.7755) (-0.7263, -14.7702) (-0.725, -14.7649) (-0.7237, -14.7597) (-0.7225, -14.7545) (-0.7213, -14.7493) (-0.7201, -14.7442) (-0.7189, -14.7392) (-0.7177, -14.7342) (-0.7166, -14.7292) (-0.7155, -14.7243) (-0.7144, -14.7194) (-0.7133, -14.7145) (-0.7123, -14.7097) (-0.7112, -14.705) (-0.7102, -14.7003) (-0.7092, -14.6956) (-0.7082, -14.691) (-0.7073, -14.6864) (-0.7064, -14.6819) (-0.7054, -14.6774) (-0.7045, -14.673) (-0.7037, -14.6686) (-0.7028, -14.6643) (-0.702, -14.66) (-0.7011, -14.6558) (-0.7003, -14.6516) (-0.6995, -14.6475) (-0.6988, -14.6434) (-0.698, -14.6394) (-0.6973, -14.6354) (-0.6966, -14.6314) (-0.6959, -14.6275) (-0.6952, -14.6237) (-0.6945, -14.6199) (-0.6939, -14.6162) (-0.6933, -14.6125) (-0.6926, -14.6089) (-0.6921, -14.6054) (-0.6915, -14.6018) (-0.6909, -14.5984) (-0.6904, -14.595) (-0.6898, -14.5916) (-0.6893, -14.5883) (-0.6888, -14.5851) (-0.6883, -14.5819) (-0.6879, -14.5788) (-0.6874, -14.5757) (-0.687, -14.5727) (-0.6866, -14.5698) (-0.6862, -14.5669) (-0.6858, -14.5641) (-0.6854, -14.5613) (-0.685, -14.5586) (-0.6847, -14.5559) (-0.6844, -14.5533) (-0.684, -14.5508) (-0.6837, -14.5484) (-0.6834, -14.546) (-0.6832, -14.5436) (-0.6829, -14.5414) (-0.6826, -14.5392) (-0.6824, -14.537) (-0.6822, -14.5349) (-0.6819, -14.5329) (-0.6817, -14.531) (-0.6815, -14.5291) (-0.6814, -14.5273) (-0.6812, -14.5256) (-0.681, -14.5239) (-0.6809, -14.5223) (-0.6807, -14.5208) (-0.6806, -14.5193) (-0.6805, -14.518) (-0.6804, -14.5167) (-0.6803, -14.5154) (-0.6802, -14.5143) (-0.6801, -14.5132) (-0.68, -14.5122) (-0.6799, -14.5112) (-0.6799, -14.5104) (-0.6798, -14.5096) (-0.6798, -14.5089) (-0.6797, -14.5083) (-0.6797, -14.5078) (-0.6797, -14.5074) (-0.6797, -14.5072) (-0.6796, -14.507) (-0.6796, -14.5069) knots -1 -1 -1 -1 -1 -1 -0.99583333 -0.99166667 -0.9875 -0.98333333 -0.97916667 -0.975 -0.97083333 -0.96666667 -0.9625 -0.95833333 -0.95416667 -0.95 -0.94583333 -0.94166667 -0.9375 -0.93333333 -0.92916667 -0.925 -0.92083333 -0.91666667 -0.9125 -0.90833333 -0.90416667 -0.9 -0.89583333 -0.89166667 -0.8875 -0.88333333 -0.87916667 -0.875 -0.87083333 -0.86666667 -0.8625 -0.85833333 -0.85416667 -0.85 -0.84583333 -0.84166667 -0.8375 -0.83333333 -0.82916667 -0.825 -0.82083333 -0.81666667 -0.8125 -0.80833333 -0.80416667 -0.8 -0.79583333 -0.79166667 -0.7875 -0.78333333 -0.77916667 -0.775 -0.77083333 -0.76666667 -0.7625 -0.75833333 -0.75416667 -0.75 -0.74583333 -0.74166667 -0.7375 -0.73333333 -0.72916667 -0.725 -0.72083333 -0.71666667 -0.7125 -0.70833333 -0.70416667 -0.7 -0.69583333 -0.69166667 -0.6875 -0.68333333 -0.67916667 -0.675 -0.67083333 -0.66666667 -0.6625 -0.65833333 -0.65416667 -0.65 -0.64583333 -0.64166667 -0.6375 -0.63333333 -0.62916667 -0.625 -0.62083333 -0.61666667 -0.6125 -0.60833333 -0.60416667 -0.6 -0.59583333 -0.59166667 -0.5875 -0.58333333 -0.57916667 -0.575 -0.57083333 -0.56666667 -0.5625 -0.55833333 -0.55416667 -0.55 -0.54583333 -0.54166667 -0.5375 -0.53333333 -0.52916667 -0.525 -0.52083333 -0.51666667 -0.5125 -0.50833333 -0.50416667 -0.5 -0.49583333 -0.49166667 -0.4875 -0.48333333 -0.47916667 -0.475 -0.47083333 -0.46666667 -0.4625 -0.45833333 -0.45416667 -0.45 -0.44583333 -0.44166667 -0.4375 -0.43333333 -0.42916667 -0.425 -0.42083333 -0.41666667 -0.4125 -0.40833333 -0.40416667 -0.4 -0.39583333 -0.39166667 -0.3875 -0.38333333 -0.37916667 -0.375 -0.37083333 -0.36666667 -0.3625 -0.35833333 -0.35416667 -0.35 -0.34583333 -0.34166667 -0.3375 -0.33333333 -0.32916667 -0.325 -0.32083333 -0.31666667 -0.3125 -0.30833333 -0.30416667 -0.3 -0.29583333 -0.29166667 -0.2875 -0.28333333 -0.27916667 -0.275 -0.27083333 -0.26666667 -0.2625 -0.25833333 -0.25416667 -0.25 -0.24583333 -0.24166667 -0.2375 -0.23333333 -0.22916667 -0.225 -0.22083333 -0.21666667 -0.2125 -0.20833333 -0.20416667 -0.2 -0.19583333 -0.19166667 -0.1875 -0.18333333 -0.17916667 -0.175 -0.17083333 -0.16666667 -0.1625 -0.15833333 -0.15416667 -0.15 -0.14583333 -0.14166667 -0.1375 -0.13333333 -0.12916667 -0.125 -0.12083333 -0.11666667 -0.1125 -0.10833333 -0.10416667 -0.1 -0.09583333 -0.09166667 -0.0875 -0.08333333 -0.07916667 -0.075 -0.07083333 -0.06666667 -0.0625 -0.05833333 -0.05416667 -0.05 -0.04583333 -0.04166667 -0.0375 -0.03333333 -0.02916667 -0.025 -0.02083333 -0.01666667 -0.0125 -0.00833333 -0.00416667 0 0 0 0 0 0
  arc A24 (11.0419, 11.5792) -> (10.3616, 12.1917) centre (0, 0) ccw
  line L54 (0.6796, -14.5063) -> (0.6796, -14.5069)
  spline S18 degree 5 poles (-14.3564, -2.1923) (-14.3565, -2.1923) (-14.3566, -2.1923) (-14.3569, -2.1924) (-14.3572, -2.1924) (-14.3578, -2.1925) (-14.3584, -2.1926) (-14.3591, -2.1928) (-14.3598, -2.1929) (-14.3607, -2.193) (-14.3616, -2.1932) (-14.3626, -2.1934) (-14.3637, -2.1936) (-14.3648, -2.1938) (-14.366, -2.194) (-14.3673, -2.1943) (-14.3687, -2.1945) (-14.3701, -2.1948) (-14.3716, -2.1951) (-14.3732, -2.1954) (-14.3748, -2.1958) (-14.3765, -2.1961) (-14.3783, -2.1965) (-14.3801, -2.1969) (-14.382, -2.1973) (-14.384, -2.1977) (-14.386, -2.1982) (-14.3882, -2.1986) (-14.3903, -2.1991) (-14.3925, -2.1996) (-14.3948, -2.2002) (-14.3972, -2.2007) (-14.3996, -2.2013) (-14.4021, -2.2018) (-14.4046, -2.2025) (-14.4072, -2.2031) (-14.4099, -2.2037) (-14.4126, -2.2044) (-14.4154, -2.2051) (-14.4182, -2.2058) (-14.4211, -2.2065) (-14.424, -2.2072) (-14.427, -2.208) (-14.4301, -2.2088) (-14.4332, -2.2096) (-14.4364, -2.2104) (-14.4396, -2.2113) (-14.4429, -2.2122) (-14.4462, -2.2131) (-14.4496, -2.214) (-14.453, -2.2149) (-14.4565, -2.2159) (-14.46, -2.2169) (-14.4636, -2.2179) (-14.4673, -2.2189) (-14.4709, -2.22) (-14.4747, -2.2211) (-14.4785, -2.2222) (-14.4823, -2.2233) (-14.4862, -2.2244) (-14.4901, -2.2256) (-14.4941, -2.2268) (-14.4981, -2.228) (-14.5022, -2.2292) (-14.5063, -2.2305) (-14.5105, -2.2318) (-14.5147, -2.2331) (-14.519, -2.2344) (-14.5233, -2.2358) (-14.5277, -2.2372) (-14.5321, -2.2386) (-14.5365, -2.24) (-14.541, -2.2414) (-14.5455, -2.2429) (-14.5501, -2.2444) (-14.5547, -2.2459) (-14.5594, -2.2475) (-14.5641, -2.2491) (-14.5688, -2.2507) (-14.5736, -2.2523) (-14.5784, -2.2539) (-14.5833, -2.2556) (-14.5882, -2.2573) (-14.5932, -2.259) (-14.5981, -2.2608) (-14.6032, -2.2626) (-14.6082, -2.2644) (-14.6133, -2.2662) (-14.6185, -2.268) (-14.6237, -2.2699) (-14.6289, -2.2718) (-14.6342, -2.2737) (-14.6395, -2.2757) (-14.6448, -2.2776) (-14.6502, -2.2796) (-14.6556, -2.2817) (-14.661, -2.2837) (-14.6665, -2.2858) (-14.672, -2.2879) (-14.6776, -2.29) (-14.6832, -2.2922) (-14.6888, -2.2944) (-14.6945, -2.2966) (-14.7002, -2.2988) (-14.7059, -2.3011) (-14.7117, -2.3034) (-14.7175, -2.3057) (-14.7233, -2.308) (-14.7292, -2.3104) (-14.7351, -2.3128) (-14.741, -2.3152) (-14.747, -2.3176) (-14.753, -2.3201) (-14.759, -2.3226) (-14.7651, -2.3251) (-14.7712, -2.3277) (-14.7773, -2.3302) (-14.7835, -2.3328) (-14.7897, -2.3355) (-14.7959, -2.3381) (-14.8022, -2.3408) (-14.8084, -2.3435) (-14.8148, -2.3463) (-14.8211, -2.349) (-14.8275, -2.3518) (-14.8339, -2.3546) (-14.8403, -2.3575) (-14.8468, -2.3604) (-14.8533, -2.3633) (-14.8598, -2.3662) (-14.8663, -2.3691) (-14.8729, -2.3721) (-14.8795, -2.3751) (-14.8862, -2.3782) (-14.8928, -2.3812) (-14.8995, -2.3843) (-14.9062, -2.3874) (-14.913, -2.3906) (-14.9198, -2.3938) (-14.9266, -2.397) (-14.9334, -2.4002) (-14.9402, -2.4034) (-14.9471, -2.4067) (-14.954, -2.41) (-14.9609, -2.4134) (-14.9679, -2.4167) (-14.9749, -2.4201) (-14.9819, -2.4236) (-14.9889, -2.427) (-14.996, -2.4305) (-15.0031, -2.434) (-15.0102, -2.4375) (-15.0173, -2.4411) (-15.0245, -2.4447) (-15.0316, -2.4483) (-15.0388, -2.4519) (-15.0461, -2.4556) (-15.0533, -2.4593) (-15.0606, -2.463) (-15.0679, -2.4668) (-15.0752, -2.4706) (-15.0825, -2.4744) (-15.0899, -2.4782) (-15.0973, -2.4821) (-15.1047, -2.486) (-15.1121, -2.4899) (-15.1196, -2.4939) (-15.1271, -2.4978) (-15.1346, -2.5018) (-15.1421, -2.5059) (-15.1496, -2.5099) (-15.1572, -2.514) (-15.1648, -2.5182) (-15.1724, -2.5223) (-15.18, -2.5265) (-15.1876, -2.5307) (-15.1953, -2.5349) (-15.203, -2.5392) (-15.2107, -2.5435) (-15.2184, -2.5478) (-15.2262, -2.5522) (-15.2339, -2.5565) (-15.2417, -2.5609) (-15.2495, -2.5654) (-15.2574, -2.5698) (-15.2652, -2.5743) (-15.2731, -2.5788) (-15.2809, -2.5834) (-15.2888, -2.588) (-15.2968, -2.5926) (-15.3047, -2.5972) (-15.3126, -2.6019) (-15.3206, -2.6065) (-15.3286, -2.6113) (-15.3366, -2.616) (-15.3446, -2.6208) (-15.3527, -2.6256) (-15.3607, -2.6304) (-15.3688, -2.6353) (-15.3769, -2.6402) (-15.385, -2.6451) (-15.3931, -2.65) (-15.4013, -2.655) (-15.4094, -2.66) (-15.4176, -2.665) (-15.4258, -2.6701) (-15.434, -2.6752) (-15.4422, -2.6803) (-15.4505, -2.6855) (-15.4587, -2.6906) (-15.467, -2.6958) (-15.4753, -2.7011) (-15.4836, -2.7063) (-15.4919, -2.7116) (-15.5002, -2.7169) (-15.5086, -2.7223) (-15.517, -2.7277) (-15.5253, -2.7331) (-15.5337, -2.7385) (-15.5421, -2.744) (-15.5505, -2.7494) (-15.559, -2.755) (-15.5674, -2.7605) (-15.5759, -2.7661) (-15.5844, -2.7717) (-15.5929, -2.7773) (-15.6014, -2.783) (-15.6099, -2.7887) (-15.6184, -2.7944) (-15.6269, -2.8002) (-15.6355, -2.8059) (-15.6441, -2.8117) (-15.6526, -2.8176) (-15.6612, -2.8234) (-15.6698, -2.8293) (-15.6785, -2.8353) (-15.6871, -2.8412) (-15.6957, -2.8472) (-15.7044, -2.8532) (-15.713, -2.8592) (-15.7217, -2.8653) (-15.7287, -2.8702) (-15.7339, -2.8738) (-15.7374, -2.8763) (-15.7391, -2.8775) knots 0 0 0 0 0 0 0.00416667 0.00833333 0.0125 0.01666667 0.02083333 0.025 0.02916667 0.03333333 0.0375 0.04166667 0.04583333 0.05 0.05416667 0.05833333 0.0625 0.06666667 0.07083333 0.075 0.07916667 0.08333333 0.0875 0.09166667 0.09583333 0.1 0.10416667 0.10833333 0.1125 0.11666667 0.12083333 0.125 0.12916667 0.13333333 0.1375 0.14166667 0.14583333 0.15 0.15416667 0.15833333 0.1625 0.16666667 0.17083333 0.175 0.17916667 0.18333333 0.1875 0.19166667 0.19583333 0.2 0.20416667 0.20833333 0.2125 0.21666667 0.22083333 0.225 0.22916667 0.23333333 0.2375 0.24166667 0.24583333 0.25 0.25416667 0.25833333 0.2625 0.26666667 0.27083333 0.275 0.27916667 0.28333333 0.2875 0.29166667 0.29583333 0.3 0.30416667 0.30833333 0.3125 0.31666667 0.32083333 0.325 0.32916667 0.33333333 0.3375 0.34166667 0.34583333 0.35 0.35416667 0.35833333 0.3625 0.36666667 0.37083333 0.375 0.37916667 0.38333333 0.3875 0.39166667 0.39583333 0.4 0.40416667 0.40833333 0.4125 0.41666667 0.42083333 0.425 0.42916667 0.43333333 0.4375 0.44166667 0.44583333 0.45 0.45416667 0.45833333 0.4625 0.46666667 0.47083333 0.475 0.47916667 0.48333333 0.4875 0.49166667 0.49583333 0.5 0.50416667 0.50833333 0.5125 0.51666667 0.52083333 0.525 0.52916667 0.53333333 0.5375 0.54166667 0.54583333 0.55 0.55416667 0.55833333 0.5625 0.56666667 0.57083333 0.575 0.57916667 0.58333333 0.5875 0.59166667 0.59583333 0.6 0.60416667 0.60833333 0.6125 0.61666667 0.62083333 0.625 0.62916667 0.63333333 0.6375 0.64166667 0.64583333 0.65 0.65416667 0.65833333 0.6625 0.66666667 0.67083333 0.675 0.67916667 0.68333333 0.6875 0.69166667 0.69583333 0.7 0.70416667 0.70833333 0.7125 0.71666667 0.72083333 0.725 0.72916667 0.73333333 0.7375 0.74166667 0.74583333 0.75 0.75416667 0.75833333 0.7625 0.76666667 0.77083333 0.775 0.77916667 0.78333333 0.7875 0.79166667 0.79583333 0.8 0.80416667 0.80833333 0.8125 0.81666667 0.82083333 0.825 0.82916667 0.83333333 0.8375 0.84166667 0.84583333 0.85 0.85416667 0.85833333 0.8625 0.86666667 0.87083333 0.875 0.87916667 0.88333333 0.8875 0.89166667 0.89583333 0.9 0.90416667 0.90833333 0.9125 0.91666667 0.92083333 0.925 0.92916667 0.93333333 0.9375 0.94166667 0.94583333 0.95 0.95416667 0.95833333 0.9625 0.96666667 0.97083333 0.975 0.97916667 0.98333333 0.9875 0.99166667 0.99583333 1 1 1 1 1 1
  line L55 (5.2796, -13.5292) -> (5.2794, -13.5286)
  line L56 (11.2355, 9.202) -> (11.235, 9.2016)
  line L57 (9.7765, 9.6687) -> (10.3255, 10.2117)
  circle A25 centre (-7.0711, 7.0711) radius 1.7
  line L58 (7.9768, 12.1353) -> (7.9771, 12.1359)